Support Chassis  IN (Autodesk Fusion 360 design; units mm, degrees)
Autodesk Fusion 360 part; units mm, degrees
sketch "Sketch1" plane through (0, 0, 0) normal (0, 0, 1) x (1, 0, 0)
  line L0 (-75, 60.9) -> (75, 60.9)
  line L1 (75, 60.9) -> (75, -60.9)
  line L2 (75, -60.9) -> (-75, -60.9)
  line L3 (-75, -60.9) -> (-75, 60.9)
  line L4 (-75, 60.9) -> (75, -60.9) construction
  line L5 (75, 60.9) -> (-75, -60.9) construction
  line L6 (75, -40.9) -> (-75, -40.9)
  line L7 (-75, -40.9) -> (-75, 40.9)
  line L8 (-75, 40.9) -> (75, 40.9)
  line L9 (75, 40.9) -> (75, -40.9)
  line L10 (75, -40.9) -> (-75, 40.9) construction
  line L11 (-75, -40.9) -> (75, 40.9) construction
  line L12 (0, 0) -> (0, 60.9) construction
  line L13 (-75, 60.9) -> (75, 40.9) construction
  line L14 (0, 50.9) -> (-75, 50.9) construction
  line L15 (0, 50.9) -> (75, 50.9) construction
  line L16 (-2.1, 53.4) -> (-2.1, 48.4)
  arc A0 (-2.1, 48.4) -> (2.1, 48.4) centre (0, 48.4) ccw
  line L17 (2.1, 48.4) -> (2.1, 53.4)
  arc A1 (2.1, 53.4) -> (-2.1, 53.4) centre (0, 53.4) ccw
  line L18 (0, 53.4) -> (0, 48.4) construction
  arc A2 (-57.9, 53.4) -> (-62.1, 53.4) centre (-60, 53.4) ccw
  line L19 (-62.1, 53.4) -> (-62.1, 48.4)
  arc A3 (-62.1, 48.4) -> (-57.9, 48.4) centre (-60, 48.4) ccw
  line L20 (-57.9, 48.4) -> (-57.9, 53.4)
  arc A4 (62.1, 53.4) -> (57.9, 53.4) centre (60, 53.4) ccw
  line L21 (57.9, 53.4) -> (57.9, 48.4)
  arc A5 (57.9, 48.4) -> (62.1, 48.4) centre (60, 48.4) ccw
  line L22 (62.1, 48.4) -> (62.1, 53.4)
  line L23 (-75, 0) -> (75, 0) construction
  arc A6 (-62.1, -53.4) -> (-57.9, -53.4) centre (-60, -53.4) ccw
  line L24 (-62.1, -53.4) -> (-62.1, -48.4)
  arc A7 (-57.9, -48.4) -> (-62.1, -48.4) centre (-60, -48.4) ccw
  line L25 (-57.9, -48.4) -> (-57.9, -53.4)
  arc A8 (-2.1, -53.4) -> (2.1, -53.4) centre (0, -53.4) ccw
  line L26 (-2.1, -53.4) -> (-2.1, -48.4)
  line L27 (2.1, -48.4) -> (2.1, -53.4)
  arc A9 (2.1, -48.4) -> (-2.1, -48.4) centre (0, -48.4) ccw
  arc A10 (57.9, -53.4) -> (62.1, -53.4) centre (60, -53.4) ccw
  line L28 (57.9, -53.4) -> (57.9, -48.4)
  line L29 (62.1, -48.4) -> (62.1, -53.4)
  arc A11 (62.1, -48.4) -> (57.9, -48.4) centre (60, -48.4) ccw
  line L30 (-40, -20) -> (40, -20)
  arc A12 (40, -20) -> (40, 20) centre (40, 0) ccw
  line L31 (40, 20) -> (-40, 20)
  arc A13 (-40, 20) -> (-40, -20) centre (-40, 0) ccw
  line L32 (-40, 0) -> (40, 0) construction
  dimension "d1" = 121.8
  dimension "d2" = 150
  dimension "d3" = 81.8
  dimension "d13" = 4.2
  dimension "d14" = 5
  dimension "d22" = 60
  dimension "d23" = 0
  dimension "d24" = 40
  dimension "d25" = 80
  constraint perpendicular L0 L1
  constraint parallel L0 L2
  constraint perpendicular L6 L7
  constraint parallel L6 L8
  constraint horizontal L6
  constraint coincident L1 L6.start
  constraint midpoint L0 L12.end
  constraint midpoint L13 L14.start
  constraint coincident L3 L14.end
  constraint perpendicular L3 L14
  constraint coincident L1 L15.end
  constraint perpendicular L1 L15
  constraint tangent L16 A0
  constraint tangent A0 L17
  constraint parallel L16 L17
  constraint tangent L17 A1
  constraint tangent L16 A1
  constraint perpendicular L14 L18
  constraint coincident L12.start L4
  constraint midpoint L12.start L4
  constraint midpoint L12.start L5
  constraint midpoint L12.start L10
  constraint midpoint L12.start L11
  constraint coincident L12.start origin
  constraint coincident L12 A1.centre
  constraint midpoint L3 L23.start
  constraint midpoint L1 L23.end
  constraint symmetric L16.start L23 A8.start
  constraint symmetric L16.end L23 L26.end
  constraint symmetric A0.end L23 L27.start
  constraint symmetric L17.end L23 A8.end
  constraint symmetric A0 L23 A9
  constraint symmetric A1 L23 A8
  constraint symmetric A2.start L23 A6.end
  constraint symmetric A2.end L23 A6.start
  constraint symmetric A2 L23 A6
  constraint symmetric L19.end L23 L24.end
  constraint symmetric A3.end L23 A7.start
  constraint symmetric A3 L23 A7
  constraint symmetric A4.start L23 A10.end
  constraint symmetric A4.end L23 A10.start
  constraint symmetric A4 L23 A10
  constraint symmetric L21.end L23 L28.end
  constraint symmetric A5.end L23 L29.start
  constraint symmetric A5 L23 A11
  constraint tangent L30 A12
  constraint tangent A12 L31
  constraint parallel L30 L31
  constraint tangent L31 A13
  constraint tangent L30 A13
  constraint parallel L23 L32
  constraint midpoint L32 L12.start
  measures "d1" distance of L0.start L2.end
  measures "d2" distance of L0.start L0.end
  measures "d3" distance of L6.end L7.end
  measures "d13" diameter of A0
  measures "d14" distance of A1.centre A0.centre
  measures "d24" diameter of A12
  measures "d25" distance of A13.centre A12.centre
extrude "Extrude1" add sketch "Sketch1" along normal blind 19.8 contours L1 L3 L6 L7 L8 L9
extrude "Extrude2" add sketch "Sketch1" against normal blind 3
sketch "Sketch2" plane through (0, 0, 19.8) normal (0, 0, 1) x (-1, 0, 0)
  circle A0 centre (-19.4856, -7.95) radius 2.1
  circle A1 centre (-19.4856, 14.55) radius 2.1
  circle A2 centre (0, 25.8) radius 2.1
  circle A3 centre (19.4856, 14.55) radius 2.1
  circle A4 centre (19.4856, -7.95) radius 2.1
  circle A5 centre (0, -19.2) radius 2.1
  circle A6 centre (0, 3.3) radius 4
  line L0 (-35, -40.9) -> (35, -40.9)
  line L1 (35, -40.9) -> (35, 40.9)
  line L2 (35, 40.9) -> (-35, 40.9)
  line L3 (-35, 40.9) -> (-35, -40.9)
  line L4 (6.2801, -26.4921) -> (-5.3166, -26.4921) construction
  line L5 (-5.3166, -26.4921) -> (-5.3166, -36.4921) construction
  line L6 (-5.3166, -36.4921) -> (6.2801, -36.4921) construction
  line L7 (6.2801, -36.4921) -> (6.2801, -26.4921) construction
  line L8 (11.9175, 36.5887) -> (-12.1889, 36.5887) construction
  line L9 (-12.1889, 36.5887) -> (-12.1889, 26.5887) construction
  line L10 (-12.1889, 26.5887) -> (11.9175, 26.5887) construction
  line L11 (11.9175, 26.5887) -> (11.9175, 36.5887) construction
  constraint perpendicular L4 L5
  constraint parallel L4 L6
  constraint parallel L5 L7
  constraint perpendicular L8 L9
  constraint parallel L8 L10
  constraint parallel L9 L11
extrude "Extrude3" [suppressed]
named bodies: "Support Chassis"
